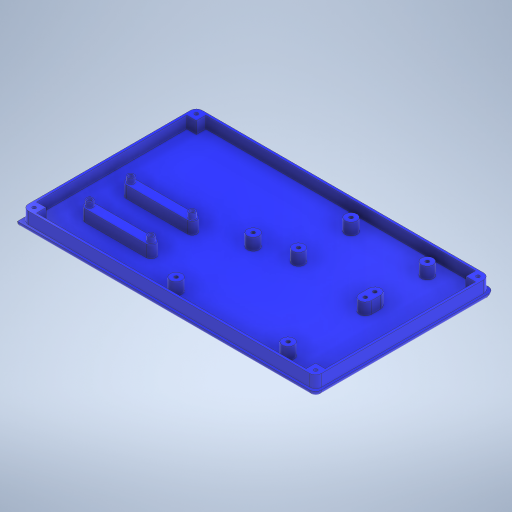
# Autodesk Inventor part: Bottom_Cover
Saved by Autodesk Inventor 2024 (Build 280153000, 153)
## iProperties
Created: 2024-05-17
Part Number: Bottom_Cover
Material: Generic
Document SubType Name: Modeling
Designer: ASUS
Density: 1 g/cm^3
Appearance: Default
Author: ASUS
Autodesk Inventor part; units mm, degrees
ref_plane "YZ Plane" through (0, 0, 0) normal (1, 0, 0) x (0, 1, 0)
ref_plane "XZ Plane" through (0, 0, 0) normal (0, 1, 0) x (-1, 0, 0)
ref_plane "XY Plane" through (0, 0, 0) normal (0, 0, 1) x (1, 0, 0)
sketch "Sketch1" plane through (0, 0, 0) normal (0, 1, 0) x (-1, 0, 0)
  line L0 (125, 75) -> (-125, 75)
  line L1 (-125, 75) -> (-125, -75)
  line L2 (-125, -75) -> (125, -75)
  line L3 (125, -75) -> (125, 75)
  line L4 (125, 75) -> (-125, -75) construction
  line L5 (-125, 75) -> (125, -75) construction
  point P0 (0, 0)
  dimension "d0" = 250
  dimension "d1" = 150
  constraints: 12 end point, 2 midpoint, 2 parallel, 1 horizontal, 1 perpendicular
  measures "d0" distance of L1.end L2.end
  measures "d1" distance of L2.end L0.start
extrude "Extrusion1" add sketch "Sketch1" along normal blind 5
sketch "Sketch2" plane through (0, 5, 0) normal (0, 1, 0) x (1, 0, 0)
  line L0 (-123, -73) -> (123, -73)
  line L1 (123, -73) -> (123, 73)
  line L2 (123, 73) -> (-123, 73)
  line L3 (-123, 73) -> (-123, -73)
  line L4 (-123, -73) -> (123, 73) construction
  line L5 (123, -73) -> (-123, 73) construction
  line L6 (-125, 75) -> (-125, -75) projected
  line L7 (125, 75) -> (-125, 75) projected
  line L8 (121, -71) -> (-121, -71)
  line L9 (-121, -71) -> (-121, 71)
  line L10 (-121, 71) -> (121, 71)
  line L11 (121, 71) -> (121, -71)
  line L12 (121, -71) -> (-121, 71) construction
  line L13 (-121, -71) -> (121, 71) construction
  point P0 (0, 0)
  dimension "d4" = 2
  dimension "d5" = 2
  dimension "d6" = 2
  dimension "d7" = 2
  constraints: 24 end point, 4 midpoint, 4 parallel, 2 horizontal, 2 perpendicular
  measures "d4" distance between parallel lines of L6 L3
  measures "d5" distance between parallel lines of L7 L2
  measures "d6" distance between parallel lines of L0 L8
  measures "d7" distance between parallel lines of L1 L11
extrude "Extrusion2" add sketch "Sketch2" along normal blind 10
sketch "Sketch3" plane through (0, 5, 0) normal (0, 1, 0) x (1, 0, 0)
  line L0 (123, 73) -> (123, -73) projected
  line L1 (123, 73) -> (113, 73)
  line L2 (113, 73) -> (113, 63)
  line L3 (113, 63) -> (123, 63)
  line L4 (123, 63) -> (123, 73)
  line L5 (123, -73) -> (113, -73)
  line L6 (113, -73) -> (113, -63)
  line L7 (113, -63) -> (123, -63)
  line L8 (123, -63) -> (123, -73)
  point P0 (0, 0)
  dimension "d10" = 10
  dimension "d11" = 10
  dimension "d12" = 10
  dimension "d13" = 10
  constraints: 16 end point, 4 parallel, 2 horizontal, 2 perpendicular
  measures "d10" distance of L2.end L3.end
  measures "d11" distance of L1.end L2.end
  measures "d12" distance of L6.end L7.end
  measures "d13" distance of L5.end L6.end
extrude "Extrusion3" add sketch "Sketch3" along normal blind 10
mirror "Mirror1" about plane through (0, 0, 0) normal (1, 0, 0) of "Extrusion3"
sketch "Sketch4" plane through (0, 15, 0) normal (0, 1, 0) x (1, 0, 0)
  circle A0 centre (118, 68) radius 1.5
  line L0 (113, 71) -> (113, 63) projected
  line L1 (113, 63) -> (121, 63) projected
  circle A1 centre (118, -68) radius 1.5
  line L2 (121, -63) -> (113, -63) projected
  line L3 (113, -63) -> (113, -71) projected
  point P0 (0, 0)
  point P1 (113, 67)
  dimension "d16" = 3
  dimension "d17" = 5
  dimension "d18" = 5
  dimension "d19" = 3
  dimension "d20" = 5
  dimension "d21" = 5
  constraints: 2 centre point, 1 midpoint
  measures "d16" diameter of A0
  measures "d17" horizontal distance of point (113, 67) A0.centre
  measures "d18" distance from line of L1 A0.centre
  measures "d19" diameter of A1
  measures "d20" distance from line of L2 A1.centre
  measures "d21" distance from line of A1.centre L3
extrude "Extrusion4" cut sketch "Sketch4" against normal through all
mirror "Mirror2" about plane through (0, 0, 0) normal (1, 0, 0) of "Extrusion4"
sketch "Sketch5" plane through (0, 0, 0) normal (0, -1, 0) x (1, 0, 0)
  circle A0 centre (117.9421, 68) radius 2.5
  circle A1 centre (118, 68) radius 1.5 projected
  circle A2 centre (118, -68) radius 2.5
  circle A3 centre (118, -68) radius 1.5 projected
  point P0 (0, 0)
  dimension "d24" = 5
  dimension "d25" = 0
  dimension "d26" = 5
  dimension "d27" = 0
  constraints: 2 centre point
  measures "d24" diameter of A0
  measures "d25" vertical distance of A0.centre A1.centre
  measures "d26" diameter of A2
  measures "d27" distance of A3.centre A2.centre
extrude "Extrusion5" cut sketch "Sketch5" against normal blind 10 contours A0 | A1 | A2 | A3
mirror "Mirror3" about plane through (0, 0, 0) normal (1, 0, 0) of "Extrusion5"
fillet "Fillet2" radius 5 4 edges at (-123, 10, -73) (123, 10, -73) (-123, 10, 73) (123, 10, 73)
sketch "Sketch7" plane through (0, 0, 0) normal (0, -1, 0) x (1, 0, 0)
  circle A0 centre (110, 60) radius 5
  line L0 (125, 75) -> (125, -75) projected
  line L1 (-125, 75) -> (125, 75) projected
  circle A1 centre (110, -60) radius 5
  line L2 (125, -75) -> (-125, -75) projected
  point P0 (0, 0)
  dimension "d32" = 10
  dimension "d33" = 15
  dimension "d34" = 15
  dimension "d35" = 10
  dimension "d36" = 15
  dimension "d37" = 15
  constraints: 2 centre point
  measures "d32" diameter of A0
  measures "d33" distance from line of L0 A0.centre
  measures "d34" distance from line of L1 A0.centre
  measures "d35" diameter of A1
  measures "d36" distance from line of L0 A1.centre
  measures "d37" distance from line of L2 A1.centre
extrude "Extrusion6" add sketch "Sketch7" along normal blind 10
fillet "Fillet3" radius 5 2 edges at (105, -10, 60) (105, -10, -60)
mirror "Mirror4" about plane through (0, 0, 0) normal (1, 0, 0) of "Extrusion6", "Fillet3"
fillet "Fillet4" radius 5 2 edges at (125, 2.5, 75) (125, 2.5, -75)
fillet "Fillet5" radius 5 5 edges at (-2.5, 0, -75) (123.5355, 0, -73.5355) (125, 0, 0) (123.5355, 0, 73.5355) (-2.5, 0, 75)
sketch "Sketch17" plane through (0, 5, 0) normal (0, 1, 0) x (1, 0, 0)
  circle A0 centre (86, -59) radius 5
  circle A1 centre (-7.974, -59) radius 5
  arc A2 (81, 5.612) -> (91, 5.612) centre (86, 5.612) ccw
  circle A3 centre (-7.974, 5.612) radius 5
  circle A4 centre (86, 57.65) radius 5
  circle A5 centre (22.048, 13.612) radius 5
  circle A6 centre (160.8835, 117.8481) radius 5
  circle A7 centre (22.048, 57.65) radius 5
  arc A8 (91, 13.612) -> (81, 13.612) centre (86, 13.612) ccw
  line L0 (113, -71) -> (-113, -71) projected
  line L1 (121, 63) -> (121, -63) projected
  line L2 (91, 13.612) -> (91, 5.612)
  line L3 (81, 5.612) -> (81, 13.612)
  point P0 (0, 0)
  dimension "d117" = 10
  dimension "d118" = 10
  dimension "d119" = 10
  dimension "d120" = 10
  dimension "d121" = 10
  dimension "d122" = 10
  dimension "d123" = 10
  dimension "d124" = 10
  dimension "d125" = 10
  dimension "d126" = 93.974
  dimension "d127" = 8
  dimension "d128" = 64.612
  dimension "d129" = 44.038
  dimension "d130" = 63.952
  dimension "d131" = 12
  dimension "d132" = 35
  constraints: 9 centre point, 5 vertical alignment, 4 end point, 4 horizontal alignment, 4 point on circle, 1 tangent, 1 vertical
  measures "d117" diameter of A0
  measures "d118" diameter of A1
  measures "d119" diameter of A2
  measures "d120" diameter of A3
  measures "d121" diameter of A4
  measures "d122" diameter of A5
  measures "d123" diameter of A6
  measures "d124" diameter of A7
  measures "d125" diameter of A8
  measures "d126" distance of A1.centre A0.centre
  measures "d127" distance of A2.centre A8.centre
  measures "d128" distance of A0.centre A2.centre
  measures "d129" distance of A8.centre A4.centre
  measures "d130" distance of A7.centre A4.centre
  measures "d131" distance from line of L0 A0.centre
  measures "d132" distance from line of L1 A0.centre
extrude "Extrusion11" add sketch "Sketch17" along normal blind 10 contours A0 | A1 | L3 A8 L2 A2 | A3 | A4 | A5 | A7
sketch "Sketch18" plane through (0, 15, 0) normal (0, 1, 0) x (1, 0, 0)
  circle A0 centre (86, -59) radius 1.5
  circle A1 centre (-7.974, -59) radius 1.5
  circle A2 centre (86, 5.612) radius 1.5
  circle A3 centre (86, 13.612) radius 1.5
  circle A4 centre (22.048, 57.65) radius 1.5
  circle A5 centre (22.048, 13.612) radius 1.5
  circle A6 centre (-7.974, 5.612) radius 1.5
  circle A7 centre (86, 57.65) radius 1.5
  circle A8 centre (86, -59) radius 5 projected
  circle A9 centre (-7.974, -59) radius 5 projected
  arc A10 (91, 13.612) -> (81, 13.612) centre (86, 13.612) ccw projected
  arc A11 (81, 5.612) -> (91, 5.612) centre (86, 5.612) ccw projected
  circle A12 centre (86, 57.65) radius 5 projected
  circle A13 centre (22.048, 13.612) radius 5 projected
  circle A14 centre (22.048, 57.65) radius 5 projected
  circle A15 centre (-7.974, 5.612) radius 5 projected
  point P0 (0, 0)
  dimension "d135" = 3
  dimension "d136" = 3
  dimension "d137" = 3
  dimension "d138" = 3
  dimension "d139" = 3
  dimension "d140" = 3
  dimension "d141" = 3
  dimension "d142" = 3
  constraints: 8 centre point, 8 concentric
  measures "d135" diameter of A0
  measures "d136" diameter of A1
  measures "d137" diameter of A2
  measures "d138" diameter of A3
  measures "d139" diameter of A4
  measures "d140" diameter of A5
  measures "d141" diameter of A6
  measures "d142" diameter of A7
extrude "Extrusion12" cut sketch "Sketch18" against normal blind 8 contours A0 | A1 | A2 | A3 | A4 | A5 | A6 | A7
sketch "Sketch20" plane through (0, 5, 0) normal (0, 1, 0) x (1, 0, 0)
  arc A0 (-44.5, -47.5) -> (-44.5, -39.5) centre (-44.5, -43.5) ccw
  arc A1 (-96, -39.5) -> (-96, -47.5) centre (-96, -43.5) ccw
  line L0 (-44.5, -47.5) -> (-96, -47.5)
  line L1 (-96, -47.5) -> (-96, -39.5)
  line L2 (-96, -39.5) -> (-44.5, -39.5)
  line L3 (-44.5, -39.5) -> (-44.5, -47.5)
  line L4 (113, -71) -> (-113, -71) projected
  line L5 (-121, -63) -> (-121, 63) projected
  arc A2 (-44.5, -13) -> (-44.5, -5) centre (-44.5, -9) ccw
  arc A3 (-96, -5) -> (-96, -13) centre (-96, -9) ccw
  line L6 (-44.5, -13) -> (-96, -13)
  line L7 (-96, -13) -> (-96, -5)
  line L8 (-96, -5) -> (-44.5, -5)
  line L9 (-44.5, -5) -> (-44.5, -13)
  line L10 (-113, 71) -> (113, 71) projected
  point P0 (0, 0)
  dimension "d145" = 8
  dimension "d146" = 8
  dimension "d147" = 51.5
  dimension "d149" = 25
  dimension "d150" = 8
  dimension "d151" = 8
  dimension "d152" = 51.5
  dimension "d153" = 34.5
  dimension "d168" = 80
  constraints: 16 end point, 8 point on circle, 4 centre point, 4 parallel, 2 horizontal, 2 horizontal alignment, 2 midpoint, 2 perpendicular, 2 tangent, 1 vertical alignment
  measures "d145" diameter of A1
  measures "d146" diameter of A0
  measures "d147" distance of A1.centre A0.centre
  measures "d149" distance from line of L5 A1.centre
  measures "d150" diameter of A3
  measures "d151" diameter of A2
  measures "d152" distance of A3.centre A2.centre
  measures "d153" distance of A1.centre A3.centre
  measures "d168" distance from line of L10 A3.centre
extrude "Extrusion13" add sketch "Sketch20" along normal blind 10
sketch "Sketch21" plane through (0, 15, 0) normal (0, 1, 0) x (1, 0, 0)
  circle A0 centre (-44.5, -43.5) radius 2.8
  arc A1 (-44.5, -47.5) -> (-44.5, -39.5) centre (-44.5, -43.5) ccw projected
  circle A2 centre (-96, -43.5) radius 2.8
  circle A3 centre (-44.5, -9) radius 2.8
  circle A4 centre (-96, -9) radius 2.8
  arc A5 (-96, -39.5) -> (-96, -47.5) centre (-96, -43.5) ccw projected
  arc A6 (-44.5, -13) -> (-44.5, -5) centre (-44.5, -9) ccw projected
  arc A7 (-96, -5) -> (-96, -13) centre (-96, -9) ccw projected
  point P0 (0, 0)
  dimension "d156" = 5.6
  dimension "d157" = 5.6
  dimension "d158" = 5.6
  dimension "d159" = 5.6
  constraints: 4 centre point, 4 concentric
  measures "d156" diameter of A0
  measures "d157" diameter of A2
  measures "d158" diameter of A3
  measures "d159" diameter of A4
extrude "Extrusion14" add sketch "Sketch21" along normal blind 4.55
sketch "Sketch22" plane through (-44.5, 19.55, 9) normal (0, 1, 0) x (1, 0, 0)
  circle A0 centre (-51.5, -34.5) radius 1.8
  circle A1 centre (-51.5, 0) radius 1.8
  circle A2 centre (0, 0) radius 1.8
  circle A3 centre (0, -34.5) radius 1.8
  circle A4 centre (-51.5, -34.5) radius 2.8 projected
  circle A5 centre (-51.5, 0) radius 2.8 projected
  circle A6 centre (0, 0) radius 2.8 projected
  circle A7 centre (0, -34.5) radius 2.8 projected
  point P0 (44.5, 9)
  dimension "d162" = 3.6
  dimension "d163" = 3.6
  dimension "d164" = 3.6
  dimension "d165" = 3.6
  constraints: 4 centre point, 4 concentric
  measures "d162" diameter of A0
  measures "d163" diameter of A1
  measures "d164" diameter of A2
  measures "d165" diameter of A3
extrude "Extrusion15" cut sketch "Sketch22" against normal blind 10 contours A0 | A1 | A2 | A3
thread "Thread5" size "M3x0.5" class "6H" standard "ANSI Metric M Profile" full length
thread "Thread6" size "M3x0.5" class "6H" standard "ANSI Metric M Profile" full length
thread "Thread7" size "M3x0.5" class "6H" standard "ANSI Metric M Profile" full length
thread "Thread8" size "M3x0.5" class "6H" standard "ANSI Metric M Profile" full length
thread "Thread9" size "M3x0.5" class "6H" standard "ANSI Metric M Profile" full length
thread "Thread10" size "M3x0.5" class "6H" standard "ANSI Metric M Profile" full length
thread "Thread11" size "M3x0.5" class "6H" standard "ANSI Metric M Profile" full length
thread "Thread12" size "M3x0.5" class "6H" standard "ANSI Metric M Profile" full length
body "Solid1"
